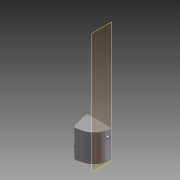
# Autodesk Inventor part: VoltageSource
Saved by Autodesk Inventor 2012 SP2 (Build 160219200, 219)
## iProperties
Created: 2014-02-09
Part Number: VoltageSource
Material: Default
Document SubType Name: Modeling
Designer: 1
Density: 1 g/cm^3
Author: 1
Autodesk Inventor part; units mm, degrees
ref_plane "XZ Plane" through (0, 0, 0) normal (0, 1, 0) x (-1, 0, 0)
ref_plane "XY Plane" through (0, 0, 0) normal (0, 0, 1) x (1, 0, 0)
sketch "Sketch1" plane through (0, 0, 0) normal (0, 0, 1) x (1, 0, 0)
  line L0 (125.1975, -635.9781) -> (-63.4844, -635.9781)
  line L1 (-63.4844, -635.9781) -> (-63.4844, -848.7632)
  line L2 (-63.4844, -848.7632) -> (125.1975, -848.7632)
  line L3 (125.1975, -848.7632) -> (125.1975, -635.9781)
  point P0 (0, 0)
  constraints: 8 end point, 2 parallel, 1 horizontal, 1 perpendicular
extrude "Extrusion1" add sketch "Sketch1" along normal blind 144.4625
sketch "Sketch2" plane through (-63.4844, -848.7632, 0) normal (0, -1, 0) x (1, 0, 0)
  line L0 (188.6819, 144.4625) -> (0, 144.4625) projected
  line L1 (0, 0) -> (0, 144.4625) projected
  line L2 (188.6819, 0) -> (188.6819, 144.4625) projected
  line L3 (0, 17.8487) -> (30.8457, 144.4625)
  line L4 (30.8457, 144.4625) -> (188.6819, 109.8581)
  point P0 (63.4844, 0)
  constraints: 4 end point, 3 point on line
extrude "Extrusion2" cut sketch "Sketch2" against normal through all
sketch "Sketch3" plane through (-63.4844, -848.7632, 17.8487) normal (-0.9715834, 0, 0.2366975) x (0.2366975, 0, 0.9715834)
  line L0 (0, 0) -> (0, 212.7851) projected
  circle A0 centre (61.7012, 50.3399) radius 23.1304
  line L1 (15.4405, 202.9114) -> (25.6712, 202.9114)
  line L2 (25.6712, 202.9114) -> (25.6712, 176.2225)
  line L3 (25.6712, 176.2225) -> (15.4405, 176.2225)
  line L4 (15.4405, 176.2225) -> (15.4405, 202.9114)
  line L5 (15.4405, 172.4314) -> (25.6712, 172.4314)
  line L6 (25.6712, 172.4314) -> (25.6712, 145.7425)
  line L7 (25.6712, 145.7425) -> (15.4405, 145.7425)
  line L8 (15.4405, 145.7425) -> (15.4405, 172.4314)
  line L9 (15.4405, 141.9514) -> (25.6712, 141.9514)
  line L10 (25.6712, 141.9514) -> (25.6712, 115.2625)
  line L11 (25.6712, 115.2625) -> (15.4405, 115.2625)
  line L12 (15.4405, 115.2625) -> (15.4405, 141.9514)
  point P0 (-2.3149, 848.7632)
  dimension "d6" = 30.48
  constraints: 24 end point, 2 parallel, 1 centre point, 1 horizontal, 1 perpendicular, 1 vertical, 16 other
  measures "d6" distance of L1.start L5.start
extrude "Extrusion3" add sketch "Sketch3" along normal blind 12.7
sketch "Sketch4" plane through (-61.219, -798.4232, 80.8026) normal (-0.9715834, 0, 0.2366975) x (0.2366975, 0, 0.9715834)
  circle A0 centre (0, 0) radius 23.1304 projected
  point P0 (-64.0161, 798.4232)
extrude "Extrusion4" add sketch "Sketch4" along normal blind 12.7
sketch "Sketch5" plane through (-63.4844, -848.7632, 17.8487) normal (-0.9715834, 0, 0.2366975) x (0.2366975, 0, 0.9715834)
  circle A0 centre (61.7012, 50.3399) radius 23.1304 projected
  circle A1 centre (61.7012, 50.3399) radius 29.0734 construction
  circle A2 centre (61.7012, 50.3399) radius 43.7714 construction
  line L0 (61.7012, 50.3399) -> (82.0253, 11.5731) construction
  arc A3 (94.4221, 21.2663) -> (38.4943, 67.8529) centre (67.5786, 45.9046) ccw
  line L1 (75.2007, 24.5906) -> (94.4221, 21.2663)
  arc A4 (75.2007, 24.5906) -> (38.4943, 67.8529) centre (61.7012, 50.3399) ccw
  point P0 (-2.3149, 848.7632)
  dimension "d15" = 87.5428
  dimension "d16" = 58.1469
  constraints: 8 point on circle, 4 centre point, 4 end point, 3 coincident, 1 point on line, 1 tangent
  measures "d15" diameter of A2
  measures "d16" diameter of A1
extrude "Extrusion5" cut sketch "Sketch5" along normal mid plane 12.7 contours L1 A4 A3
fillet "Fillet1" radius 130.175 1 edges at (125.1975, -742.3706, 109.8581)
fillet "Fillet2" radius 4.7625 1 edges at (-79.033, -798.4232, 61.3356)
chamfer "Chamfer1" distance 14.2875 angle 45 1 edges at (-32.6387, -742.3706, 144.4625)
ref_plane "Work Plane1" through (119.0625, 0, 0) normal (1, 0, 0) x (0, 1, 0)
sketch "Sketch6" plane through (119.0625, 0, 0) normal (1, 0, 0) x (0, 1, 0)
  circle A0 centre (-684.0193, 29.4352) radius 9.6445
  point P0 (0, 0)
  constraints: 1 centre point
extrude "Extrusion6" add sketch "Sketch6" along normal blind 12.7
body "Solid1"
